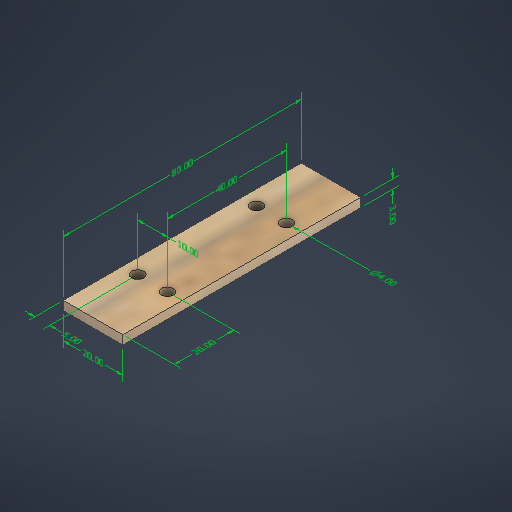
# Autodesk Inventor part: Soporte_Techo
Saved by Autodesk Inventor 2026.2 (Build 302298000, 298)
## iProperties
Created: 2026-03-25
Part Number: Soporte_Techo
Material: Genérico
Document SubType Name: Sheet Metal
Designer: yahir
Density: 1 g/cm^3
Sheet Metal Rule: Por defecto_mm
Appearance: Valor por defecto
Author: yahir
Autodesk Inventor part; units mm, degrees
ref_plane "YZ Plane" through (0, 0, 0) normal (1, 0, 0) x (0, 1, 0)
ref_plane "XZ Plane" through (0, 0, 0) normal (0, 1, 0) x (-1, 0, 0)
ref_plane "XY Plane" through (0, 0, 0) normal (0, 0, 1) x (1, 0, 0)
sketch "Boceto1" plane through (0, 0, 0) normal (0, 1, 0) x (-1, 0, 0)
  line L0 (10, 0) -> (10, -40)
  line L1 (10, -40) -> (-10, -40)
  line L2 (-10, -40) -> (-10, 40)
  line L3 (-10, 40) -> (10, 40)
  line L4 (10, 40) -> (10, 0)
  line L5 (0, 0) -> (0, 20)
  line L6 (0, 20) -> (5, 20)
  line L7 (0, 0) -> (0, -20)
  line L8 (0, -20) -> (5, -20)
  line L9 (0, 20) -> (-5, 20)
  line L10 (0, -20) -> (-5, -20)
  circle A0 centre (5, 20) radius 2
  circle A1 centre (5, -20) radius 2
  circle A2 centre (-5, -20) radius 2
  circle A3 centre (-5, 20) radius 2
  dimension "d1" = 40
  dimension "d2" = 20
  dimension "d3" = 80
  dimension "d5" = 20
  dimension "d6" = 5
  dimension "d7" = 20
  dimension "d8" = 5
  dimension "d9" = 5
  dimension "d10" = 4
  dimension "d11" = 4
  dimension "d12" = 4
  dimension "d13" = 4
  constraints: 22 end point, 6 perpendicular, 4 centre point, 4 coincident, 2 point on line, 2 vertical, 1 horizontal
  measures "d1" distance of L0.start L0.end
  measures "d2" distance of L0.end L1.end
  measures "d3" distance of L1.end L2.end
  measures "d5" distance of L5.start L5.end
  measures "d6" distance of L5.end L6.end
  measures "d7" distance of L5.start L7.end
  measures "d8" distance of L5.end L9.end
  measures "d9" distance of L7.end L10.end
  measures "d10" diameter of A0
  measures "d11" diameter of A1
  measures "d12" diameter of A2
  measures "d13" diameter of A3
extrude "Extrusión1" add sketch "Boceto1" along normal blind 3
equation "\"Radio_pliegue\" = Grosor"
equation "\"Anchura_desahogo_plegado\" = Grosor"
equation "\"Profundidad_desahogo_plegado\" = 0.5 * Grosor"
equation "\"Tamaño_destalonado\" = 4 * Grosor"
equation "\"Remanente_mínimo\" = 2 * Grosor"
equation "\"Radiodetransición\" = Radio_pliegue"
equation "\"Tamaño_de_radio_de_Jacobi\" = Radio_pliegue"
equation "\"TamañoSeparación\" = Grosor"
equation "\"Grosor\" = 0.5"
